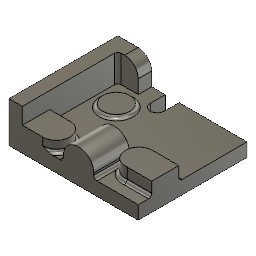
_ass 3.197890e5-097f-4753-abc8-cf540231f4e6 (Autodesk Fusion 360 design; units mm, degrees)
Autodesk Fusion 360 part; units mm, degrees
sketch "Sketch1" plane through (0, 0, 0) normal (0, 1, 0) x (1, 0, 0)
  line L0 (60.325, 50.8) -> (-60.325, 50.8)
  line L1 (-60.325, 50.8) -> (-60.325, -50.8)
  line L2 (-60.325, -50.8) -> (60.325, -50.8)
  line L3 (60.325, -50.8) -> (60.325, 50.8)
  line L4 (60.325, 50.8) -> (-60.325, -50.8) construction
  line L5 (-60.325, 50.8) -> (60.325, -50.8) construction
  dimension "d1" = 120.65
  dimension "d5" = 101.6
extrude "Extrude1" add sketch "Sketch1" along normal blind 12.7
sketch "Sketch2" plane through (0, 12.7, 0) normal (0, 1, 0) x (-1, 0, 0)
  line L0 (-60.325, 50.8) -> (-60.325, -50.8)
  line L1 (-60.325, -50.8) -> (60.325, -50.8)
  line L2 (60.325, -50.8) -> (60.325, 50.8)
  line L3 (60.325, 50.8) -> (-60.325, 50.8)
  line L4 (15.875, -50.8) -> (15.875, -36.576)
  line L5 (3.175, -50.8) -> (3.175, -36.576)
  arc A0 (15.875, -36.576) -> (3.175, -36.576) centre (9.525, -36.576) ccw
extrude "Extrude2" cut sketch "Sketch2" against normal blind 40.64 contours L1 L4 L5 A0
sketch "Sketch3" plane through (0, 12.7, 0) normal (0, 1, 0) x (-1, 0, 0)
  line L0 (15.875, -36.576) -> (15.875, -50.8)
  line L1 (15.875, -50.8) -> (60.325, -50.8)
  line L2 (60.325, -50.8) -> (60.325, 50.8)
  line L3 (60.325, 50.8) -> (-60.325, 50.8)
  line L4 (-60.325, 50.8) -> (-60.325, -50.8)
  line L5 (-60.325, -50.8) -> (3.175, -50.8)
  line L6 (3.175, -50.8) -> (3.175, -36.576)
  arc A0 (15.875, -36.576) -> (3.175, -36.576) centre (9.525, -36.576) ccw
  line L7 (-60.325, 38.1806) -> (-37.465, 38.1806)
  arc A1 (-37.465, 12.9972) -> (-37.465, 38.1806) centre (-35.8103, 25.5889) ccw
  line L8 (-37.465, 12.9972) -> (-60.325, 12.9972)
  dimension "d14" = 22.86
  dimension "d16" = 12.7
  measures "d16" radius of A1
extrude "Extrude3" add sketch "Sketch3" along normal blind 12.7 contours L4 L7 A1 L8
sketch "Sketch4" plane through (0, 0, 50.8) normal (0, 0, 1) x (1, 0, 0)
  line L0 (-60.325, 0) -> (60.325, 0)
  line L1 (60.325, 0) -> (60.325, 12.7)
  line L2 (60.325, 12.7) -> (-60.325, 12.7)
  line L3 (-60.325, 12.7) -> (-60.325, 0)
  line L4 (-15.875, 12.7) -> (-3.175, 12.7)
  line L5 (-9.525, 12.7) -> (-9.525, 17.526)
  line L6 (18.923, 12.7) -> (18.923, 17.526)
  arc A0 (18.923, 17.526) -> (-9.525, 17.526) centre (4.699, 17.526) ccw
extrude "Extrude4" add sketch "Sketch4" against normal blind 33.274 contours L2 L4 L5 L6 A0
sketch "Sketch5" plane through (0, 0, 0) normal (0, -1, 0) x (1, 0, 0)
  line L0 (-15.875, -50.8) -> (-15.875, -36.576)
  arc A0 (-3.175, -36.576) -> (-15.875, -36.576) centre (-9.525, -36.576) ccw
  line L1 (-3.175, -36.576) -> (-3.175, -50.8)
  line L2 (-3.175, -50.8) -> (60.325, -50.8)
  line L3 (60.325, -50.8) -> (60.325, 50.8)
  line L4 (60.325, 50.8) -> (-60.325, 50.8)
  line L5 (-60.325, 50.8) -> (-60.325, -50.8)
  line L6 (-60.325, -50.8) -> (-15.875, -50.8)
  line L7 (-60.325, -50.8) -> (18.923, -50.8)
  arc A1 (9.271, -38.1) -> (28.575, -38.1) centre (18.923, -38.1) ccw
  arc A2 (28.432, -13.9451) -> (9.414, -13.9451) centre (18.923, -12.2899) ccw
  line L8 (9.414, -13.9451) -> (9.271, -38.1)
  line L9 (28.432, -13.9451) -> (28.575, -38.1)
extrude "Extrude5" cut sketch "Sketch5" against normal blind 6.35 contours A1 A2 L8 L9
fillet "Fillet1" radius 3.048 5 edges at (18.923, 12.7, 34.163) (48.895, 12.7, 38.1806) (23.1103, 12.7, 25.5889) (48.895, 12.7, 12.9972) (-9.525, 12.7, 34.163)
sketch "Sketch6" plane through (0, 12.7, 0) normal (0, 1, 0) x (-1, 0, 0)
  line L0 (12.573, 50.8) -> (12.573, 17.526)
  line L1 (12.573, 17.526) -> (-21.971, 17.526)
  line L2 (-21.971, 17.526) -> (-21.971, 18.0741)
  arc A0 (-37.6537, 9.9492) -> (-21.971, 18.0741) centre (-35.8103, 25.5889) ccw
  line L3 (-37.6537, 9.9492) -> (-60.325, 9.9492)
  line L4 (-60.325, 9.9492) -> (-60.325, -50.8)
  line L5 (-60.325, -50.8) -> (3.175, -50.8)
  line L6 (3.175, -50.8) -> (3.175, -36.576)
  arc A1 (15.875, -36.576) -> (3.175, -36.576) centre (9.525, -36.576) ccw
  line L7 (15.875, -36.576) -> (15.875, -50.8)
  line L8 (15.875, -50.8) -> (60.325, -50.8)
  line L9 (60.325, -50.8) -> (60.325, 50.8)
  line L10 (60.325, 50.8) -> (12.573, 50.8)
  circle A2 centre (28.575, -17.78) radius 12.7
  dimension "d36" = 25.4
  dimension "d38" = 33.02
  dimension "d39" = 31.75
  measures "d36" diameter of A2
  measures "d38" distance of L8
extrude "Extrude6" add sketch "Sketch6" along normal blind 3.048 contours A2
fillet "Fillet2" radius 3.048 1 edges at (-16.7344, 12.7, -13.1875)
sketch "Sketch7" plane through (0, 12.7, 0) normal (0, 1, 0) x (-1, 0, 0)
  line L0 (12.573, 50.8) -> (12.573, 17.526)
  line L1 (12.573, 17.526) -> (-21.971, 17.526)
  line L2 (-21.971, 17.526) -> (-21.971, 18.0741)
  arc A0 (-37.6537, 9.9492) -> (-21.971, 18.0741) centre (-35.8103, 25.5889) ccw
  line L3 (-37.6537, 9.9492) -> (-60.325, 9.9492)
  line L4 (-60.325, 9.9492) -> (-60.325, -50.8)
  line L5 (-60.325, -50.8) -> (3.175, -50.8)
  line L6 (3.175, -50.8) -> (3.175, -36.576)
  arc A1 (15.875, -36.576) -> (3.175, -36.576) centre (9.525, -36.576) ccw
  line L7 (15.875, -36.576) -> (15.875, -50.8)
  line L8 (15.875, -50.8) -> (60.325, -50.8)
  line L9 (60.325, -50.8) -> (60.325, 50.8)
  line L10 (60.325, 50.8) -> (12.573, 50.8)
  circle A2 centre (28.575, -17.78) radius 15.748
  line L11 (60.325, -50.8) -> (47.625, -50.8)
  line L12 (47.625, -50.8) -> (47.625, 50.8)
  line L13 (47.625, 50.8) -> (60.325, 50.8)
  line L14 (60.325, 50.8) -> (60.325, -50.8)
  line L15 (47.625, 25.4) -> (28.575, 25.4)
  arc A3 (28.575, 50.8) -> (28.575, 25.4) centre (28.575, 38.1) ccw
  line L16 (47.625, 50.8) -> (28.575, 50.8)
  dimension "d43" = 12.7
  dimension "d44" = 19.05
  dimension "d45" = 19.05
  dimension "d46" = 12.7
  measures "d46" radius of A3
extrude "Extrude7" add sketch "Sketch7" along normal blind 10.16 contours L10 L12 L15 A3 L16
fillet "Fillet3" radius 3.048 2 edges at (-38.1, 12.7, 25.4) (-15.875, 12.7, 38.1)
sketch "Sketch8" plane through (0, 12.7, 0) normal (0, 1, 0) x (-1, 0, 0)
  arc A0 (19.2632, 50.8) -> (28.575, 22.352) centre (28.575, 38.1) ccw
  line L0 (19.2632, 50.8) -> (12.573, 50.8)
  line L1 (12.573, 50.8) -> (12.573, 17.526)
  line L2 (12.573, 17.526) -> (-21.971, 17.526)
  line L3 (-21.971, 17.526) -> (-21.971, 18.0741)
  arc A1 (-37.6537, 9.9492) -> (-21.971, 18.0741) centre (-35.8103, 25.5889) ccw
  line L4 (-37.6537, 9.9492) -> (-60.325, 9.9492)
  line L5 (-60.325, 9.9492) -> (-60.325, -50.8)
  line L6 (-60.325, -50.8) -> (3.175, -50.8)
  line L7 (3.175, -50.8) -> (3.175, -36.576)
  arc A2 (15.875, -36.576) -> (3.175, -36.576) centre (9.525, -36.576) ccw
  line L8 (15.875, -36.576) -> (15.875, -50.8)
  line L9 (15.875, -50.8) -> (60.325, -50.8)
  line L10 (60.325, -50.8) -> (60.325, 50.8)
  line L11 (60.325, 50.8) -> (47.625, 50.8)
  line L12 (47.625, 50.8) -> (47.625, 22.352)
  line L13 (47.625, 22.352) -> (28.575, 22.352)
  circle A3 centre (28.575, -17.78) radius 15.748
  line L14 (60.325, -50.8) -> (41.275, -50.8)
  line L15 (41.275, -50.8) -> (41.275, -38.1)
  line L16 (41.275, -38.1) -> (60.325, -38.1)
  line L17 (60.325, -38.1) -> (60.325, -50.8)
  dimension "d51" = 12.7
  dimension "d53" = 19.05
extrude "Extrude8" add sketch "Sketch8" along normal blind 25.4 contours L9 L10 L14 L15 L16 L17
sketch "Sketch9" plane through (0, 12.7, 0) normal (0, 1, 0) x (-1, 0, 0)
  circle A0 centre (28.575, -17.78) radius 15.748
  line L0 (41.275, -50.8) -> (41.275, -38.1)
  line L1 (41.275, -38.1) -> (60.325, -38.1)
  line L2 (60.325, -38.1) -> (60.325, 50.8)
  line L3 (60.325, 50.8) -> (47.625, 50.8)
  line L4 (47.625, 50.8) -> (47.625, 22.352)
  line L5 (47.625, 22.352) -> (28.575, 22.352)
  arc A1 (19.2632, 50.8) -> (28.575, 22.352) centre (28.575, 38.1) ccw
  line L6 (19.2632, 50.8) -> (12.573, 50.8)
  line L7 (12.573, 50.8) -> (12.573, 17.526)
  line L8 (12.573, 17.526) -> (-21.971, 17.526)
  line L9 (-21.971, 17.526) -> (-21.971, 18.0741)
  arc A2 (-37.6537, 9.9492) -> (-21.971, 18.0741) centre (-35.8103, 25.5889) ccw
  line L10 (-37.6537, 9.9492) -> (-60.325, 9.9492)
  line L11 (-60.325, 9.9492) -> (-60.325, -50.8)
  line L12 (-60.325, -50.8) -> (3.175, -50.8)
  line L13 (3.175, -50.8) -> (3.175, -36.576)
  arc A3 (15.875, -36.576) -> (3.175, -36.576) centre (9.525, -36.576) ccw
  line L14 (15.875, -36.576) -> (15.875, -50.8)
  line L15 (15.875, -50.8) -> (41.275, -50.8)
  line L16 (41.275, -38.1) -> (28.575, -38.1)
  line L17 (28.575, -38.1) -> (28.575, -50.8)
  line L18 (28.575, -50.8) -> (41.275, -50.8)
  line L19 (41.275, -50.8) -> (41.275, -38.1)
  dimension "d56" = 12.7
extrude "Extrude9" add sketch "Sketch9" along normal blind 12.7 contours L0 L15 L16 L17 L18 L19
sketch "Sketch10" plane through (0, 0, -38.1) normal (0, 0, 1) x (1, 0, 0)
  line L0 (-60.325, 12.7) -> (-28.575, 12.7)
  line L1 (-28.575, 12.7) -> (-28.575, 25.4)
  line L2 (-28.575, 25.4) -> (-41.275, 25.4)
  line L3 (-41.275, 25.4) -> (-41.275, 38.1)
  line L4 (-41.275, 38.1) -> (-60.325, 38.1)
  line L5 (-60.325, 38.1) -> (-60.325, 12.7)
  arc A0 (-28.575, 25.4) -> (-41.275, 38.1) centre (-41.275, 25.4) ccw
extrude "Extrude10" add sketch "Sketch10" against normal blind 12.7 contours L2 L3 A0
sketch "Sketch11" plane through (0, 12.7, 0) normal (0, 1, 0) x (-1, 0, 0)
  line L0 (28.575, -50.8) -> (28.575, -38.1)
  line L1 (28.575, -38.1) -> (60.325, -38.1)
  line L2 (60.325, -38.1) -> (60.325, 50.8)
  line L3 (60.325, 50.8) -> (47.625, 50.8)
  line L4 (47.625, 50.8) -> (47.625, 22.352)
  line L5 (47.625, 22.352) -> (28.575, 22.352)
  arc A0 (19.2632, 50.8) -> (28.575, 22.352) centre (28.575, 38.1) ccw
  line L6 (19.2632, 50.8) -> (12.573, 50.8)
  line L7 (12.573, 50.8) -> (12.573, 17.526)
  line L8 (12.573, 17.526) -> (-21.971, 17.526)
  line L9 (-21.971, 17.526) -> (-21.971, 18.0741)
  arc A1 (-37.6537, 9.9492) -> (-21.971, 18.0741) centre (-35.8103, 25.5889) ccw
  line L10 (-37.6537, 9.9492) -> (-60.325, 9.9492)
  line L11 (-60.325, 9.9492) -> (-60.325, -50.8)
  line L12 (-60.325, -50.8) -> (3.175, -50.8)
  line L13 (3.175, -50.8) -> (3.175, -36.576)
  arc A2 (15.875, -36.576) -> (3.175, -36.576) centre (9.525, -36.576) ccw
  line L14 (15.875, -36.576) -> (15.875, -50.8)
  line L15 (15.875, -50.8) -> (28.575, -50.8)
  circle A3 centre (28.575, -17.78) radius 15.748
  line L16 (60.325, -38.1) -> (47.625, -38.1)
  line L17 (47.625, -38.1) -> (47.625, 50.8)
  line L18 (47.625, 50.8) -> (60.325, 50.8)
  line L19 (60.325, 50.8) -> (60.325, -38.1)
  dimension "d61" = 12.7
extrude "Extrude11" add sketch "Sketch11" along normal blind 25.4 contours L1 L2 L3 L4 L16 L17 L18 L19
fillet "Fillet4" radius 3.048 1 edges at (-47.625, 25.4, -38.1)
